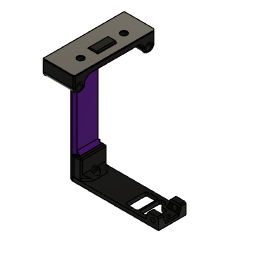
Dock_MK011 (Autodesk Fusion 360 design; units mm, degrees)
Autodesk Fusion 360 part; units mm, degrees
note: some values were not read from the file. Set by a fixed rule: which sketch regions a step uses; which face or edge a step refers to.
sketch "Sketch1" plane through (0, 0, 0) normal (1, 0, 0) x (0, 1, 0) in component "Main"
  circle A0 centre (-28, 0) radius 2.625
  circle A1 centre (28, 0) radius 2.625
  line L0 (28, 0) -> (-28, 0) construction
  line L1 (-32.75, 8.5) -> (32.75, 8.5)
  circle A2 centre (28, 0) radius 4.75
  circle A3 centre (-28, 0) radius 4.75
  line L2 (32.75, 8.5) -> (32.75, 0)
  line L3 (-32.75, 8.5) -> (-32.75, 0)
  line L4 (23.25, 0) -> (23.25, 4)
  line L5 (23.25, 4) -> (-23.25, 4)
  line L6 (-23.25, 4) -> (-23.25, 0)
  line L7 (0, 1.75) -> (0, 22.5) construction
  dimension "d1" = 5.25
  dimension "d2" = 5.25
  dimension "d3" = 56
  dimension "d4" = 8.5
  dimension "d5" = 9.5
  dimension "d6" = 9.5
  dimension "d7" = 4.5
  constraint coincident A1.centre L0.start
  constraint coincident A0.centre L0.end
  constraint horizontal L0
  constraint midpoint origin L0
  constraint horizontal L1
  constraint coincident A2 L2.end
  constraint tangent A2 L2
  constraint coincident A3 L3.end
  constraint tangent A3 L3
  constraint vertical L3
  constraint vertical L2
  constraint coincident L0 L4.start
  constraint coincident A2 L4.start
  constraint parallel L0 L5
  constraint coincident L0 L6.end
  constraint coincident A3 L6.end
  constraint symmetric L4 L6 L7
  constraint tangent A3 L6
  measures "d1" diameter of A0
  measures "d2" diameter of A1
  measures "d3" distance of A1.centre A0.centre
  measures "d4" distance of L0 L1
  measures "d5" diameter of A2
  measures "d6" diameter of A3
  measures "d7" distance of L1 L5
extrude "Extrude1" add sketch "Sketch1" along normal blind 25 makes body 1 in component "Main"
chamfer "Chamfer1" distance 3 angle 45 2 edges at (12.5, -23.25, 4) (12.5, 23.25, 4) on bodies 1 in component "Main"
sketch "Sketch2" plane through (0, 0, 8.5) normal (0, 0, 1) x (-1, 0, 0) in component "Main"
  line L0 (0, -32.75) -> (0, 32.75)
  line L1 (0, 32.75) -> (-25, 32.75)
  line L2 (-25, 32.75) -> (-25, -32.75)
  line L3 (-25, -32.75) -> (0, -32.75)
  line L4 (-15, 32.75) -> (-15, -32.75) construction
  circle A0 centre (-15, -17.5) radius 2.65
  circle A1 centre (-15, 17.5) radius 2.65
  line L5 (0, 0) -> (-15, 0) construction
  circle A2 centre (-15, 17.5) radius 4.75
  circle A3 centre (-15, -17.5) radius 4.75
  dimension "d12" = 5.3
  dimension "d13" = 5.3
  dimension "d16" = 15
  dimension "d19" = 35
  dimension "d20" = 9.5
  dimension "d21" = 9.5
  constraint coincident L4 A0.centre
  constraint coincident L4 A1.centre
  constraint coincident L5.start origin
  constraint midpoint L4 L5.end
  constraint symmetric A0 A1 L5
  constraint concentric A1 A2
  constraint concentric A0 A3
  measures "d12" diameter of A0
  measures "d13" diameter of A1
  measures "d16" distance of L0 L4
  measures "d19" distance of A0.centre A1.centre
  measures "d20" diameter of A2
  measures "d21" diameter of A3
extrude "Extrude3" cut sketch "Sketch2" against normal blind 19 from surface at -3 contours A2 | A3 bodies 1 in component "Main"
extrude "Extrude2" cut sketch "Sketch2" against normal blind 19 contours A0 | A1 bodies 1 in component "Main"
sketch "Sketch3" plane through (0, 0, 8.5) normal (0, 0, 1) x (-1, 0, 0) in component "Main"
  circle A0 centre (-15, -17.5) radius 2.65
  circle A1 centre (-15, 17.5) radius 2.65
  line L0 (0, -32.75) -> (0, 32.75)
  line L1 (0, 32.75) -> (-25, 32.75)
  line L2 (-25, 32.75) -> (-25, -32.75)
  line L3 (-25, -32.75) -> (0, -32.75)
  line L4 (-15, -17.5) -> (-15, 17.5) construction
  line L5 (-11.1, 7.5) -> (-18.9, 7.5)
  line L6 (-18.9, 7.5) -> (-18.9, -7.5)
  line L7 (-18.9, -7.5) -> (-11.1, -7.5)
  line L8 (-11.1, -7.5) -> (-11.1, 7.5)
  line L9 (0, 0) -> (-15, 0) construction
  line L10 (-15, -7.5) -> (-15, 7.5) construction
  point P0 (-15, -7.5)
  point P1 (-15, 7.5)
  point P2 (-15, 0)
  dimension "d25" = 7.8
  dimension "d26" = 15
  constraint coincident A0.centre L4.start
  constraint coincident A1.centre L4.end
  constraint horizontal L5
  constraint vertical L6
  constraint horizontal L7
  constraint vertical L8
  constraint midpoint L7 P0
  constraint midpoint L5 P1
  constraint coincident L4 P0
  constraint coincident L9.start origin
  constraint midpoint L4 P2
  constraint coincident P0 L10.start
  constraint coincident P1 L10.end
  constraint midpoint L10 P2
  constraint coincident L9 P2
  measures "d25" distance of L6.end L7.end
  measures "d26" distance of L5.end L6.end
extrude "Extrude4" add sketch "Sketch3" along normal blind 2 contours L5 L6 L7 L8 bodies 1 in component "Main"
chamfer "Chamfer2" distance 1 angle 45 2 edges at (18.9, 0, 10.5) (11.1, 0, 10.5) on bodies 1 in component "Main"
sketch "Sketch5" plane through (0, 0, 8.5) normal (0, 0, 1) x (-1, 0, 0) in component "Main"
  line L0 (-11.1, -7.5) -> (-18.9, -7.5)
  line L1 (-18.9, -7.5) -> (-18.9, 7.5)
  line L2 (-18.9, 7.5) -> (-11.1, 7.5)
  line L3 (-11.1, 7.5) -> (-11.1, -7.5)
  circle A0 centre (-15, -17.5) radius 2.65
  circle A1 centre (-15, 17.5) radius 2.65
  line L4 (0, -32.75) -> (0, 32.75)
  line L5 (0, 32.75) -> (-25, 32.75)
  line L6 (-25, 32.75) -> (-25, -32.75)
  line L7 (-25, -32.75) -> (0, -32.75)
  circle A2 centre (-4, -6.5) radius 2.5 construction
  circle A3 centre (-4, 6.5) radius 2.5 construction
  line L8 (0, 0) -> (-11.1, 0) construction
  circle A4 centre (-4, -6.5) radius 1.65
  circle A5 centre (-4, 6.5) radius 1.65
  dimension "d43" = 5
  dimension "d44" = 5
  dimension "d45" = 13
  dimension "d46" = 3.3
  dimension "d47" = 3.3
  dimension "d48" = 4
  constraint coincident L8.start origin
  constraint midpoint L3 L8.end
  constraint symmetric A2.centre A3.centre L8
  constraint concentric A2 A4
  constraint concentric A3 A5
  measures "d43" diameter of A2
  measures "d44" diameter of A3
  measures "d45" distance of A2.centre A3.centre
  measures "d46" diameter of A4
  measures "d47" diameter of A5
  measures "d48" distance of L4 A3.centre
extrude "Extrude6" cut sketch "Sketch5" against normal up to surface (4.5 mm away) contours A4 | A5 bodies 1 in component "Main"
sketch "Sketch6" plane through (0, 0, 8.5) normal (0, 0, 1) x (-1, 0, 0) in component "Main"
  circle A0 centre (-4, -6.5) radius 1.65
  circle A1 centre (-4, 6.5) radius 1.65
  line L0 (-11.1, -7.5) -> (-18.9, -7.5)
  line L1 (-18.9, -7.5) -> (-18.9, 7.5)
  line L2 (-18.9, 7.5) -> (-11.1, 7.5)
  line L3 (-11.1, 7.5) -> (-11.1, -7.5)
  circle A2 centre (-15, -17.5) radius 2.65
  circle A3 centre (-15, 17.5) radius 2.65
  line L4 (0, -32.75) -> (0, 32.75)
  line L5 (0, 32.75) -> (-25, 32.75)
  line L6 (-25, 32.75) -> (-25, -32.75)
  line L7 (-25, -32.75) -> (0, -32.75)
  circle A4 centre (-4, -6.5) radius 3.35
  circle A5 centre (-4, 6.5) radius 3.35
  dimension "d52" = 6.7
  dimension "d53" = 6.7
  constraint concentric A0 A4
  constraint concentric A1 A5
  measures "d52" diameter of A4
  measures "d53" diameter of A5
extrude "Extrude7" cut sketch "Sketch6" against normal blind 3.5 contours A4 | A5 bodies 1 in component "Main"
sketch "Sketch1 (2)" plane through (0, 0, 4) normal (0, 0, -1) x (1, 0, 0) in component "Wiper_arm"
  circle A0 centre (4, -6.5) radius 1.65
  circle A1 centre (4, 6.5) radius 1.65
  arc A2 (11.127, 20.25) -> (18.873, 20.25) centre (15, 17.5) ccw
  line L0 (11.127, 20.25) -> (0, 20.25)
  line L1 (0, 20.25) -> (0, -20.25)
  line L2 (0, -20.25) -> (11.127, -20.25)
  arc A3 (18.873, -20.25) -> (11.127, -20.25) centre (15, -17.5) ccw
  line L3 (18.873, -20.25) -> (25, -20.25)
  line L4 (25, -20.25) -> (25, 20.25)
  line L5 (25, 20.25) -> (18.873, 20.25)
  line L6 (0, 10.5) -> (8, 10.5)
  line L7 (8, 10.5) -> (8, -10.5)
  line L8 (8, -10.5) -> (0, -10.5)
  line L9 (0, -10.5) -> (0, 10.5)
  circle A4 centre (4, -6.5) radius 2.25
  circle A5 centre (4, 6.5) radius 2.25
  dimension "d57" = 4.5
  dimension "d58" = 4.5
  dimension "d59" = 4
  dimension "d60" = 4
  dimension "d61" = 4
  constraint horizontal L6
  constraint vertical L7
  constraint horizontal L8
  constraint vertical L9
  constraint coincident L1 L6.start
  constraint concentric A0 A4
  constraint concentric A1 A5
  measures "d57" diameter of A4
  measures "d58" diameter of A5
  measures "d59" distance of L7 A1.centre
  measures "d60" distance of L6 A1.centre
  measures "d61" distance of L8 A0.centre
extrude "Extrude1'" add sketch "Sketch1 (2)" along normal blind 5 from surface at 0.2 separate body contours L1 L6 L7 L8 L9 makes body 2 in component "Wiper_arm"
sketch "Sketch2 (2)" plane through (0, -10.5, 0) normal (0, -1, 0) x (1, 0, 0) in component "Wiper_arm"
  line L0 (8, 3.8) -> (0, 3.8)
  line L1 (0, 3.8) -> (0, -1.2)
  line L2 (0, -1.2) -> (8, -1.2)
  line L3 (8, -1.2) -> (8, 3.8)
  line L4 (0, -1.2) -> (0, -86.5)
  line L5 (3, -3.0199) -> (3, -86.5)
  line L6 (8, -1.2) -> (3, -3.0199)
  line L7 (0, -86.5) -> (3, -86.5)
  line L8 (0.65, 8.5) -> (7.35, 8.5)
  line L9 (0.65, 8.5) -> (7.35, 8.5)
  line L10 (11.1, 8.5) -> (18.9, 8.5)
  line L11 (18.9, 8.5) -> (11.1, 8.5)
  line L12 (12.35, 8.5) -> (17.65, 8.5)
  line L13 (12.35, 8.5) -> (17.65, 8.5)
  line L14 (0, 8.5) -> (25, 8.5)
  line L15 (25, 8.5) -> (0, 8.5)
  dimension "d66" = 110
  dimension "d67" = 3
  dimension "d69" = 95
  constraint coincident L1.end L2.start
  constraint vertical L4
  constraint vertical L5
  constraint horizontal L7
  constraint coincident L2.end L3.start
  measures "d66" angle of L5 L6
  measures "d67" distance of L4 L5
  measures "d69" distance of L7 L11
extrude "Extrude2'" add sketch "Sketch2 (2)" against normal up to surface (21 mm away) contours L2 L4 L5 L6 L7 bodies 2 in component "Wiper_arm"
chamfer "Chamfer1'" distance 2 angle 45 1 edges at (3, 0, -3.0199) on bodies 2 in component "Wiper_arm"
chamfer "Chamfer2'" distance 1 angle 45 1 edges at (8, 0, -1.2) on bodies 2 in component "Wiper_arm"
chamfer "Chamfer3" distance 2 angle 45 2 edges at (3, 10.5, -45.7599) (3, -10.5, -45.7599) on bodies 2 in component "Wiper_arm"
sketch "Sketch3 (2)" plane through (3, 0, 0) normal (1, 0, 0) x (0, 1, 0) in component "Wiper_arm"
  line L0 (-8.5, -5.0199) -> (-8.5, -86.5)
  line L1 (-8.5, -86.5) -> (8.5, -86.5)
  line L2 (8.5, -86.5) -> (8.5, -5.0199)
  line L3 (8.5, -5.0199) -> (-8.5, -5.0199)
  line L4 (0, -86.5) -> (0, -55.7891) construction
  arc A0 (-1.75, -79.5) -> (1.75, -79.5) centre (0, -79.5) ccw
  arc A1 (1.75, -73.5) -> (-1.75, -73.5) centre (0, -73.5) ccw
  line L5 (1.75, -73.5) -> (1.75, -79.5)
  line L6 (-1.75, -73.5) -> (-1.75, -79.5)
  dimension "d78" = 1.75
  dimension "d79" = 1.75
  dimension "d80" = 6
  dimension "d81" = 7
  constraint midpoint L1 L4.start
  constraint perpendicular L1 L4
  constraint coincident L4 A0.centre
  constraint coincident L4 A1.centre
  constraint vertical L6
  constraint vertical L5
  constraint tangent A1 L5
  constraint tangent A1 L6
  measures "d78" radius of A0
  measures "d79" radius of A1
  measures "d80" distance of A0.centre A1.centre
  measures "d81" distance of L1 A0.centre
extrude "Extrude3'" cut sketch "Sketch3 (2)" against normal up to surface (3 mm away) contours A0 A1 L5 L6 bodies 2 in component "Wiper_arm"
sketch "Sketch4" plane through (0, 0, 0) normal (-1, 0, 0) x (0, -1, 0) in component "Wiper_arm"
  line L0 (-1.75, -79.5) -> (-1.75, -73.5)
  arc A0 (1.75, -73.5) -> (-1.75, -73.5) centre (0, -73.5) ccw
  line L1 (1.75, -73.5) -> (1.75, -79.5)
  arc A1 (-1.75, -79.5) -> (1.75, -79.5) centre (0, -79.5) ccw
  line L2 (10.5, 3.8) -> (-10.5, 3.8)
  line L3 (-10.5, 3.8) -> (-10.5, -86.5)
  line L4 (-10.5, -86.5) -> (10.5, -86.5)
  line L5 (10.5, -86.5) -> (10.5, 3.8)
  line L6 (2.9, -71.8257) -> (0, -70.1514)
  line L7 (0, -70.1514) -> (-2.9, -71.8257)
  line L8 (-2.9, -71.8257) -> (-2.9, -75.1743)
  line L9 (-2.9, -75.1743) -> (0, -76.8486) construction
  line L10 (0, -76.8486) -> (2.9, -75.1743) construction
  line L11 (2.9, -75.1743) -> (2.9, -71.8257)
  line L12 (2.9, -77.8257) -> (0, -76.1514) construction
  line L13 (0, -76.1514) -> (-2.9, -77.8257) construction
  line L14 (-2.9, -77.8257) -> (-2.9, -81.1743)
  line L15 (-2.9, -81.1743) -> (0, -82.8486)
  line L16 (0, -82.8486) -> (2.9, -81.1743)
  line L17 (2.9, -81.1743) -> (2.9, -77.8257)
  line L18 (2.9, -77.8257) -> (2.9, -75.1743)
  line L19 (-2.9, -77.8257) -> (-2.9, -75.1743)
  point P0 (0, -73.5)
  point P1 (0, -79.5)
  dimension "d84" = 2.9
  dimension "d85" = 2.9
  constraint coincident P0 A0.centre
  constraint coincident P1 A1.centre
  constraint vertical L17
  constraint vertical L11
  measures "d84" distance of P0 L11
  measures "d85" distance of P1 L17
sketch "Sketch5 (2)" plane through (3, 0, 0) normal (1, 0, 0) x (0, 1, 0) in component "Wiper_arm"
  line L0 (1.75, -73.5) -> (1.75, -79.5)
  arc A0 (-1.75, -79.5) -> (1.75, -79.5) centre (0, -79.5) ccw
  line L1 (-1.75, -79.5) -> (-1.75, -73.5)
  arc A1 (1.75, -73.5) -> (-1.75, -73.5) centre (0, -73.5) ccw
  line L2 (-8.5, -5.0199) -> (-8.5, -86.5)
  line L3 (-8.5, -86.5) -> (8.5, -86.5)
  line L4 (8.5, -86.5) -> (8.5, -5.0199)
  line L5 (8.5, -5.0199) -> (-8.5, -5.0199)
  line L6 (-8.5, -68.5) -> (8.5, -68.5)
  dimension "d88" = 5
  constraint coincident L2 L6.start
  constraint coincident L4 L6.end
  constraint perpendicular L4 L6
  measures "d88" distance of A1.centre L6
extrude "Extrude5" add sketch "Sketch5 (2)" along normal blind 2.5 contours L2 L3 L4 L6 bodies 2 in component "Wiper_arm"
extrude "Extrude4'" cut sketch "Sketch4" against normal blind 3.5 contours L6 L7 L8 L11 L14 L15 L16 L17 L18 L19 bodies 2 in component "Wiper_arm"
chamfer "Chamfer4" distance 2.5 angle 45 1 edges at (3, 0, -68.5) on bodies 2 in component "Wiper_arm"
sketch "Sketch1 (3)" plane through (5.5, 0, 0) normal (1, 0, 0) x (0, 1, 0) in component "Wiper"
  arc A0 (-1.75, -79.5) -> (1.75, -79.5) centre (0, -79.5) ccw
  line L0 (-1.75, -79.5) -> (-1.75, -73.5)
  arc A1 (1.75, -73.5) -> (-1.75, -73.5) centre (0, -73.5) ccw
  line L1 (1.75, -73.5) -> (1.75, -79.5)
  line L2 (-8.5, -86.5) -> (8.5, -86.5)
  line L3 (8.5, -86.5) -> (8.5, -68.5)
  line L4 (8.5, -68.5) -> (-8.5, -68.5)
  line L5 (-8.5, -68.5) -> (-8.5, -86.5)
  line L6 (-10.5, -7.8761) -> (-10.5, -86.5)
  line L7 (10.5, -86.5) -> (10.5, -7.8761)
  line L8 (-10.5, -68.5) -> (10.5, -68.5)
  line L9 (10.5, -68.5) -> (10.5, -86.5)
  line L10 (10.5, -86.5) -> (-10.5, -86.5)
  line L11 (-10.5, -86.5) -> (-10.5, -68.5)
  line L12 (8.5, -68.5) -> (-8.5, -68.5)
  circle A2 centre (0, -79.5) radius 1.75
  constraint horizontal L8
  constraint vertical L9
  constraint horizontal L10
  constraint vertical L11
  constraint coincident L6 L8.start
  constraint coincident L7.start L9.end
  constraint coincident L4.end L8
  constraint concentric A0 A2
  constraint coincident A0.end A2
extrude "Extrude1''" add sketch "Sketch1 (3)" along normal blind 3 separate body contours L0 A1 L1 A2 | L2 L3 L4 L5 L8 L10 L12 | L5 L6 L8 L10 L11 | L3 L7 L8 L9 L10 makes body 3 in component "Wiper"
sketch "Sketch2 (3)" plane through (0, 0, -68.5) normal (0, 0, 1) x (-1, 0, 0) in component "Wiper"
  line L0 (-5.5, -10.5) -> (-5.5, 10.5)
  line L1 (-5.5, 10.5) -> (-8.5, 10.5)
  line L2 (-8.5, 10.5) -> (-8.5, -10.5)
  line L3 (-8.5, -10.5) -> (-5.5, -10.5)
  line L4 (-3, 8.5) -> (-5.5, 8.5)
  line L5 (-5.5, 8.5) -> (-3, 8.5)
  line L6 (-1, 10.5) -> (-3, 8.5)
  line L7 (-3, 8.5) -> (-1, 10.5)
  line L8 (-3, -8.5) -> (-5.5, -8.5)
  line L9 (-5.5, -8.5) -> (-3, -8.5)
  line L10 (-3, -8.5) -> (-1, -10.5)
  line L11 (-1, -10.5) -> (-3, -8.5)
  line L12 (-5.5, 10.5) -> (-2.6971, 10.5)
  line L13 (-2.6971, 10.5) -> (-1.8485, 11.3485)
  line L14 (-1, 10.5) -> (-1.8485, 11.3485)
  line L15 (0, 0) -> (-5.5, 0) construction
  line L16 (-3, -8.5) -> (-5.5, -8.5)
  line L17 (-5.5, -8.5) -> (-3, -8.5)
  line L18 (-3, -8.5) -> (-1, -10.5)
  line L19 (-1, -10.5) -> (-3, -8.5)
  line L20 (-2.6971, -10.5) -> (-1.8485, -11.3485)
  line L21 (-5.5, -10.5) -> (-2.6971, -10.5)
  line L22 (-1, -10.5) -> (-1.8485, -11.3485)
  dimension "d94" = 1.2
  constraint coincident L0.end L1.start
  constraint perpendicular L0 L12
  constraint parallel L6 L13
  constraint coincident L6.start L7.end
  constraint perpendicular L13 L14
  constraint coincident L15.start origin
  constraint midpoint L0 L15.end
  constraint symmetric L4.start L15 L8.start
  constraint symmetric L4.end L15 L8.end
  constraint symmetric L6.start L15 L10.end
  constraint symmetric L0.end L15 L0.start
  constraint symmetric L12.end L15 L20.start
  constraint symmetric L13.end L15 L20.end
  measures "d94" distance of L13.end L6.start
extrude "Extrude2''" add sketch "Sketch2 (3)" against normal up to surface (18 mm away) contours L0 L8 L9 L10 L11 L16 L17 L18 L19 L20 L21 L22 | L0 L4 L5 L6 L7 L12 L13 L14 bodies 3 in component "Wiper"
move_face "OffsetFaces1" offset -0.15 1 faces at (1.6667, -9.8333, -74.5) on bodies 3 in component "Wiper"
move_face "OffsetFaces2" offset -0.15 2 faces at (4.6667, 8.5, -74.5) (3.9748, -8.5, -74.5) on bodies 3 in component "Wiper"
move_face "OffsetFaces3" offset -0.2 1 faces at (5.5, 0.0436, -71.585) on bodies 3 in component "Wiper"
chamfer "Chamfer1''" distance 1 angle 45 6 edges at (8.5, 10.5, -77.5) (8.5, -10.5, -77.5) (8.5, 0, -68.5) (5.5985, -10.5, -68.5) (4.0985, 10.5, -68.5) (7, 10.5, -68.5) on bodies 3 in component "Wiper"
sketch "Sketch3 (3)" plane through (0, 0, -86.5) normal (0, 0, -1) x (1, 0, 0) in component "Wiper"
  line L0 (8.5, 9.5) -> (7.5, 10.5)
  line L1 (7.5, 10.5) -> (2.6971, 10.5)
  line L2 (2.6971, 10.5) -> (1.8485, 11.3485)
  line L3 (1.8485, 11.3485) -> (1.1061, 10.6061)
  line L4 (1.1061, 10.6061) -> (3.0621, 8.65)
  line L5 (3.0621, 8.65) -> (5.7, 8.65)
  line L6 (5.7, 8.65) -> (5.7, -8.65)
  line L7 (5.7, -8.65) -> (2.85, -8.65)
  line L8 (2.85, -8.65) -> (1, -10.5)
  line L9 (1, -10.5) -> (1.8485, -11.3485)
  line L10 (1.8485, -11.3485) -> (2.6971, -10.5)
  line L11 (2.6971, -10.5) -> (5.5, -10.5)
  line L12 (5.5, -10.5) -> (7.5, -10.5)
  line L13 (7.5, -10.5) -> (8.5, -9.5)
  line L14 (8.5, -9.5) -> (8.5, 9.5)
  line L15 (8.5, 9.5) -> (70, 9.5)
  line L16 (8.5, -9.5) -> (70, -9.5)
  line L17 (70, -9.5) -> (70, 9.5)
  line L18 (0, 2.9) -> (0, 0)
  line L19 (0, 0) -> (0, -2.9)
  line L20 (0, -2.9) -> (0, 0)
  line L21 (0, 0) -> (0, 2.9)
  line L22 (0, 10.5) -> (0, -10.5)
  line L23 (0, -10.5) -> (0, 10.5)
  line L24 (70, 11.1) -> (70, 9.5)
  line L25 (70, -9.5) -> (70, 9.5)
  line L26 (70, -11.1) -> (70, -9.5)
  line L27 (70, 11.1) -> (2.0971, 11.1)
  line L28 (70, -11.1) -> (2.0602, -11.1)
  line L29 (70, -11.1) -> (71.6, -11.1)
  line L30 (71.6, -11.1) -> (71.6, 11.1)
  line L31 (71.6, 11.1) -> (70, 11.1)
  line L32 (70, 11.1) -> (70, -11.1)
  dimension "d101" = 70
  dimension "d102" = 1.6
  dimension "d103" = 1.6
  dimension "d106" = 1.6
  constraint coincident L0.start L14.end
  constraint perpendicular L14 L15
  constraint coincident L13.end L14.start
  constraint perpendicular L14 L16
  constraint vertical L17
  constraint perpendicular L15 L25
  constraint perpendicular L16 L26
  constraint horizontal L27
  constraint vertical L24
  constraint perpendicular L26 L28
  constraint coincident L2 L27.end
  constraint horizontal L29
  constraint vertical L30
  constraint horizontal L31
  constraint vertical L32
  measures "d101" distance of L17 L22
  measures "d102" distance of L16.end L26.start
  measures "d103" distance of L15.end L24.start
  measures "d106" distance of L30 L32
extrude "Extrude3''" add sketch "Sketch3 (3)" against normal blind 3 contours L14 L15 L16 L17 L25 L32 | L0 L1 L2 L15 L24 L27 L32 | L10 L11 L12 L13 L16 L26 L28 L32 | L17 L24 L25 L26 L29 L30 L31 L32 bodies 3 in component "Wiper"
sketch "Sketch4 (2)" plane through (0, 0, -83.5) normal (0, 0, 1) x (-1, 0, 0) in component "Wiper"
  line L0 (-71.6, -11.1) -> (-2.0971, -11.1)
  line L1 (-2.0971, -11.1) -> (-2.6971, -10.5)
  line L2 (-2.6971, -10.5) -> (-5.5, -10.5)
  line L3 (-5.5, -10.5) -> (-7.5, -10.5)
  line L4 (-7.5, -10.5) -> (-8.5, -9.5)
  line L5 (-8.5, -9.5) -> (-8.5, 9.5)
  line L6 (-8.5, 9.5) -> (-7.5, 10.5)
  line L7 (-7.5, 10.5) -> (-2.6971, 10.5)
  line L8 (-2.6971, 10.5) -> (-2.0971, 11.1)
  line L9 (-2.0971, 11.1) -> (-71.6, 11.1)
  line L10 (-71.6, 11.1) -> (-71.6, -11.1)
  line L11 (-71.6, -11.1) -> (-62.6, -11.1)
  line L12 (-62.6, -11.1) -> (-62.6, -7.1)
  line L13 (-62.6, -7.1) -> (-71.6, -7.1)
  line L14 (-71.6, -7.1) -> (-71.6, -11.1)
  line L15 (-71.6, 11.1) -> (-62.6, 11.1)
  line L16 (-62.6, 11.1) -> (-62.6, 7.1)
  line L17 (-62.6, 7.1) -> (-71.6, 7.1)
  line L18 (-71.6, 7.1) -> (-71.6, 11.1)
  line L19 (-71.6, 0) -> (-66.592, 0) construction
  dimension "d107" = 4
  dimension "d108" = 9
  constraint horizontal L11
  constraint vertical L12
  constraint horizontal L13
  constraint vertical L14
  constraint coincident L0.start L10.end
  constraint horizontal L15
  constraint vertical L16
  constraint horizontal L17
  constraint vertical L18
  constraint coincident L9.end L10.start
  constraint collinear L12 L16
  constraint midpoint L10 L19.start
  constraint perpendicular L10 L19
  constraint symmetric L13 L17 L19
  measures "d107" distance of L15.end L16.end
  measures "d108" distance of L12.end L13.end
extrude "Extrude4''" add sketch "Sketch4 (2)" along normal blind 6 contours L0 L10 L11 L12 L13 L14 | L9 L10 L15 L16 L17 L18 bodies 3 in component "Wiper"
sketch "Sketch5 (3)" plane through (0, -11.1, 0) normal (0, -1, 0) x (1, 0, 0) in component "Wiper"
  line L0 (2.0971, -86.5) -> (71.6, -86.5)
  line L1 (71.6, -86.5) -> (71.6, -77.5)
  line L2 (71.6, -77.5) -> (62.6, -77.5)
  line L3 (62.6, -77.5) -> (62.6, -83.5)
  line L4 (62.6, -83.5) -> (2.0971, -83.5)
  line L5 (2.0971, -83.5) -> (2.0971, -86.5)
  circle A0 centre (67.1, -81.5) radius 1.75
  line L6 (67.1, -77.5) -> (67.1, -86.5) construction
  dimension "d111" = 3.5
  dimension "d112" = 4
  constraint midpoint L2 L6.start
  constraint coincident L0 L6.end
  constraint perpendicular L0 L6
  constraint coincident A0.centre L6
  measures "d111" diameter of A0
  measures "d112" distance of L2 A0.centre
extrude "Extrude5'" cut sketch "Sketch5 (3)" against normal up to surface (22.2 mm away) contours A0 bodies 3 in component "Wiper"
chamfer "Chamfer2''" distance 1.5 angle 65 4 edges at (67.1, 7.1, -83.5) (67.1, -7.1, -83.5) (62.6, -9.1, -83.5) (62.6, 9.1, -83.5) measured on face at (26.5333, -2.3667, -83.5) measured on face at (26.5333, -2.3667, -83.5) measured on face at (26.5333, -2.3667, -83.5) measured on face at (26.5333, -2.3667, -83.5) on bodies 3 in component "Wiper"
chamfer "Chamfer3'" distance 1 angle 45 1 edges at (71.6, 0, -83.5) on bodies 3 in component "Wiper"
sketch "Sketch6 (2)" plane through (0, 0, -83.5) normal (0, 0, 1) x (-1, 0, 0) in component "Wiper"
  line L0 (-70.6, -5.6) -> (-61.1, -5.6)
  line L1 (-61.1, -5.6) -> (-61.1, -11.1)
  line L2 (-61.1, -11.1) -> (-2.0971, -11.1)
  line L3 (-2.0971, -11.1) -> (-2.6971, -10.5)
  line L4 (-2.6971, -10.5) -> (-5.5, -10.5)
  line L5 (-5.5, -10.5) -> (-7.5, -10.5)
  line L6 (-7.5, -10.5) -> (-8.5, -9.5)
  line L7 (-8.5, -9.5) -> (-8.5, 9.5)
  line L8 (-8.5, 9.5) -> (-7.5, 10.5)
  line L9 (-7.5, 10.5) -> (-2.6971, 10.5)
  line L10 (-2.6971, 10.5) -> (-2.0971, 11.1)
  line L11 (-2.0971, 11.1) -> (-61.1, 11.1)
  line L12 (-61.1, 11.1) -> (-61.1, 5.6)
  line L13 (-61.1, 5.6) -> (-70.6, 5.6)
  line L14 (-71.6, 5.1337) -> (-71.6, -5.1337)
  line L15 (-71.6, 0) -> (-57.3301, 0) construction
  circle A0 centre (-68.1, 0) radius 1.45
  line L16 (-70.6, 5.6) -> (-70.6, -5.6)
  dimension "d117" = 2.9
  dimension "d118" = 3.5
  constraint midpoint L14 L15.start
  constraint perpendicular L14 L15
  constraint coincident L15 A0.centre
  measures "d117" diameter of A0
  measures "d118" distance of L14 A0.centre
extrude "Extrude6'" cut sketch "Sketch6 (2)" against normal up to surface (3 mm away) contours A0 bodies 3 in component "Wiper"
chamfer "Chamfer4'" distance 1 angle 45 4 edges at (62.6, 9.1, -77.5) (71.6, 9.1, -77.5) (71.6, -9.1, -77.5) (62.6, -9.1, -77.5) on bodies 3 in component "Wiper"
chamfer "Chamfer4''" distance 1 angle 45 9 edges at (25, 28, -4.75) (25, 32.75, 4.25) (25, 23.25, 0.5) (25, 21.75, 2.5) (25, 0, 4) (25, -21.75, 2.5) (25, -28, -4.75) (25, -23.25, 0.5) (25, -32.75, 4.25) on bodies 1 in component "Main"
chamfer "Chamfer5" distance 4 angle 50 1 edges at (8.5, 0, -83.5) measured on face at (8.5, -0.0436, -72.2516) on bodies 3 in component "Wiper"
sketch "Sketch1 (4)" plane through (8.5, 0, 0) normal (1, 0, 0) x (0, 1, 0)
  line L0 (1.75, -79.5) -> (9.5, -79.5)
  line L1 (9.5, -79.5) -> (9.5, -69.5)
  line L2 (9.5, -69.5) -> (-9.5, -69.5)
  line L3 (-9.5, -69.5) -> (-9.5, -79.5)
  circle A0 centre (0, -79.5) radius 3.25
  line L4 (-9.5, -79.5) -> (-1.75, -79.5)
  arc A1 (1.75, -79.5) -> (-1.75, -79.5) centre (0, -79.5) ccw
  dimension "d124" = 6.5
  measures "d124" diameter of A0
extrude "Extrude7'" cut sketch "Sketch1 (4)" along normal blind 4 contours L0 A0 L4 A1 | L0 A0 L4 A1 bodies 3 in component "Wiper"
chamfer "Chamfer6" distance 1 angle 45 2 edges at (10.3835, 7.6165, -83.5) (10.3835, -7.6165, -83.5) on bodies 3 in component "Wiper"
sketch "Sketch6 (3)" plane through (3.5, 0, 0) normal (-1, 0, 0) x (0, -1, 0) in component "Wiper_arm"
  arc A0 (1.75, -73.5) -> (-1.75, -73.5) centre (0, -73.5) ccw
  line L0 (1.75, -73.5) -> (1.75, -79.5)
  arc A1 (-1.75, -79.5) -> (1.75, -79.5) centre (0, -79.5) ccw
  line L1 (-1.75, -79.5) -> (-1.75, -73.5)
  line L2 (-2.9, -81.1743) -> (0, -82.8486)
  line L3 (0, -82.8486) -> (2.9, -81.1743)
  line L4 (2.9, -81.1743) -> (2.9, -71.8257)
  line L5 (2.9, -71.8257) -> (0, -70.1514)
  line L6 (0, -70.1514) -> (-2.9, -71.8257)
  line L7 (-2.9, -71.8257) -> (-2.9, -81.1743)
extrude "Extrude6''" add sketch "Sketch6 (3)" against normal blind 0.2 contours A0 L0 A1 L1 bodies 2 in component "Wiper_arm"
sketch "Sketch2 (4)" plane through (0, 0, 8.5) normal (0, 0, 1) x (-1, 0, 0)
  circle A0 centre (-15, 17.5) radius 2.65
  circle A1 centre (-15, -17.5) radius 2.65
  line L0 (-11.1, -7.5) -> (-18.9, -7.5)
  line L1 (-18.9, -7.5) -> (-18.9, 7.5)
  line L2 (-18.9, 7.5) -> (-11.1, 7.5)
  line L3 (-11.1, 7.5) -> (-11.1, -7.5)
  circle A2 centre (-4, -6.5) radius 3.35
  circle A3 centre (-4, 6.5) radius 3.35
  line L4 (-25, -31.75) -> (-24, -32.75)
  line L5 (-24, -32.75) -> (0, -32.75)
  line L6 (0, -32.75) -> (0, 32.75)
  line L7 (0, 32.75) -> (-24, 32.75)
  line L8 (-24, 32.75) -> (-25, 31.75)
  line L9 (-25, 31.75) -> (-25, -31.75)
extrude "Extrude1'''" add sketch "Sketch2 (4)" along normal blind 0.6 from surface at 0.2 separate body contours A2 | A3 | L4 L5 L6 L7 L8 L9 makes body 4
move_face "OffsetFaces1'" offset -0.15 4 faces at (13.7, 7.5, 8.9) (11.1, -2.5, 8.9) (18.9, 2.5, 8.9) (16.3, -7.5, 8.9) on bodies 4
sketch "Sketch3 (4)" plane through (0, 0, -83.5) normal (0, 0, 1) x (-1, 0, 0)
  line L0 (-13.267, -6.1472) -> (-13.267, 6.1472)
  line L1 (-13.267, 6.1472) -> (-8.9142, 10.5)
  line L2 (-8.9142, 10.5) -> (-2.6971, 10.5)
  line L3 (-2.6971, 10.5) -> (-2.0971, 11.1)
  line L4 (-2.0971, 11.1) -> (-61.1, 11.1)
  line L5 (-61.1, 11.1) -> (-61.1, 5.6)
  line L6 (-61.1, 5.6) -> (-70.6, 5.6)
  line L7 (-70.6, 5.6) -> (-70.6, -5.6)
  line L8 (-70.6, -5.6) -> (-61.1, -5.6)
  line L9 (-61.1, -5.6) -> (-61.1, -11.1)
  line L10 (-61.1, -11.1) -> (-2.0971, -11.1)
  line L11 (-2.0971, -11.1) -> (-2.6971, -10.5)
  line L12 (-2.6971, -10.5) -> (-5.5, -10.5)
  line L13 (-5.5, -10.5) -> (-8.9142, -10.5)
  line L14 (-8.9142, -10.5) -> (-13.267, -6.1472)
  circle A0 centre (-68.1, 0) radius 1.45
  line L15 (-64.1, -3.6) -> (-42.1, -3.6)
  line L16 (-42.1, -3.6) -> (-42.1, 3.6)
  line L17 (-42.1, 3.6) -> (-64.1, 3.6)
  line L18 (-64.1, 3.6) -> (-64.1, -3.6)
  line L19 (-58.6, -3.6) -> (-58.6, -8.6)
  line L20 (-58.6, -8.6) -> (-42.1, -8.6)
  line L21 (-42.1, -8.6) -> (-42.1, -3.6)
  line L22 (-42.1, 3.6) -> (-42.1, 8.6)
  line L23 (-42.1, 8.6) -> (-58.6, 8.6)
  line L24 (-58.6, 8.6) -> (-58.6, 3.6)
  dimension "d135" = 4
  dimension "d136" = 2
  dimension "d137" = 2
  dimension "d138" = 2.5
  dimension "d139" = 2.5
  dimension "d140" = 2.5
  dimension "d141" = 22
  constraint horizontal L15
  constraint vertical L16
  constraint horizontal L17
  constraint vertical L18
  constraint coincident L15 L19.start
  constraint perpendicular L15 L19
  constraint perpendicular L19 L20
  constraint perpendicular L17 L22
  constraint perpendicular L16 L23
  constraint coincident L17 L24.end
  constraint perpendicular L17 L24
  constraint vertical L21
  constraint collinear L19 L24
  measures "d135" distance of A0.centre L18
  measures "d136" distance of L8 L15
  measures "d137" distance of L6 L17
  measures "d138" distance of L9 L19
  measures "d139" distance of L10 L20
  measures "d140" distance of L4 L23
  measures "d141" distance of L16 L18
extrude "Extrude8" cut sketch "Sketch3 (4)" against normal up to surface (3.2 mm away) from surface at 0.2 contours L15 L16 L17 L18 | L15 L19 L20 L21 | L17 L22 L23 L24 bodies 3 in component "Wiper"
sketch "Sketch4 (3)" plane through (0, 0, -83.5) normal (0, 0, 1) x (-1, 0, 0)
  line L0 (-58.6, -3.6) -> (-64.1, -3.6)
  line L1 (-64.1, -3.6) -> (-64.1, 3.6)
  line L2 (-64.1, 3.6) -> (-58.6, 3.6)
  line L3 (-58.6, 3.6) -> (-58.6, 8.6)
  line L4 (-58.6, 8.6) -> (-42.1, 8.6)
  line L5 (-42.1, 8.6) -> (-42.1, -8.6)
  line L6 (-42.1, -8.6) -> (-58.6, -8.6)
  line L7 (-58.6, -8.6) -> (-58.6, -3.6)
  line L8 (-13.267, -6.1472) -> (-13.267, 6.1472)
  line L9 (-13.267, 6.1472) -> (-8.9142, 10.5)
  line L10 (-8.9142, 10.5) -> (-2.6971, 10.5)
  line L11 (-2.6971, 10.5) -> (-2.0971, 11.1)
  line L12 (-2.0971, 11.1) -> (-61.1, 11.1)
  line L13 (-61.1, 11.1) -> (-61.1, 5.6)
  line L14 (-61.1, 5.6) -> (-70.6, 5.6)
  line L15 (-70.6, 5.6) -> (-70.6, -5.6)
  line L16 (-70.6, -5.6) -> (-61.1, -5.6)
  line L17 (-61.1, -5.6) -> (-61.1, -11.1)
  line L18 (-61.1, -11.1) -> (-2.0971, -11.1)
  line L19 (-2.0971, -11.1) -> (-2.6971, -10.5)
  line L20 (-2.6971, -10.5) -> (-5.5, -10.5)
  line L21 (-5.5, -10.5) -> (-8.9142, -10.5)
  line L22 (-8.9142, -10.5) -> (-13.267, -6.1472)
  circle A0 centre (-68.1, 0) radius 1.45
  line L23 (-52.1, -8.6) -> (-53.3, -8.6)
  line L24 (-53.3, -8.6) -> (-53.3, 8.6)
  line L25 (-53.3, 8.6) -> (-52.1, 8.6)
  line L26 (-52.1, 8.6) -> (-52.1, -8.6)
  line L27 (-50.9885, 8.6233) -> (-52.1, -8.6) construction
  dimension "d146" = 1.2
  dimension "d151" = 6.5
  constraint horizontal L23
  constraint vertical L24
  constraint horizontal L25
  constraint vertical L26
  constraint coincident L4 L24.end
  constraint coincident L6 L23.start
  measures "d146" distance of L23.end L23.start
  measures "d151" distance of L6.end L23.start
extrude "Extrude9" add sketch "Sketch4 (3)" against normal up to surface (3 mm away) contours L4 L6 L23 L24 L25 L26 bodies 3 in component "Wiper"
chamfer "Chamfer7" distance 1 angle 45 12 edges at (42.1, 8.6, -85) (42.1, -8.6, -85) (58.6, -8.6, -85) (64.1, -3.6, -85) (58.6, -3.6, -85) (58.6, 8.6, -85) (58.6, 3.6, -85) (64.1, 3.6, -85) (53.3, 8.6, -85) (52.1, 8.6, -85) (52.1, -8.6, -85) (53.3, -8.6, -85) on bodies 3 in component "Wiper"
component "Main" placed x (1, 0, 0) y (0, 1, 0) z (0, 0, 1) at (0, 0, 0)
component "Wiper_arm" placed x (1, 0, 0) y (0, 1, 0) z (0, 0, 1) at (0, 0, 0)
component "Wiper" placed x (1, 0, 0) y (0, 1, 0) z (0, 0, 1) at (0, 0, 0)
equation "d78 = ( 3.5 / 2 ) * 1 mm"
equation "d79 = ( 3.5 / 2 ) * 1 mm"
equation "d84 = ( 5.8 / 2 ) * 1 mm"
equation "d85 = ( 5.8 / 2 ) * 1 mm"
